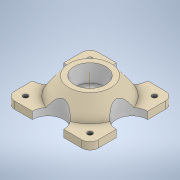
# Autodesk Inventor part: WindTurbine
Saved by Autodesk Inventor 2021 (Build 250183000, 183)
## iProperties
Created: 2022-01-11
Part Number: WindTurbine
Material: Generic
Document SubType Name: Modeling
Designer: stefi
Density: 1 g/cm^3
Appearance: Default
Author: stefi
Autodesk Inventor part; units mm, degrees
ref_plane "YZ Plane" through (0, 0, 0) normal (1, 0, 0) x (0, 1, 0)
ref_plane "XZ Plane" through (0, 0, 0) normal (0, 1, 0) x (-1, 0, 0)
ref_plane "XY Plane" through (0, 0, 0) normal (0, 0, 1) x (1, 0, 0)
sketch "Sketch1" plane through (0, 0, 0) normal (0, 1, 0) x (-1, 0, 0)
  line L0 (40.8, 50.8) -> (-40.8, 50.8)
  line L1 (-50.8, 40.8) -> (-50.8, -40.8)
  line L2 (-40.8, -50.8) -> (40.8, -50.8)
  line L3 (50.8, -40.8) -> (50.8, 40.8)
  line L4 (50.8, 50.8) -> (-50.8, -50.8) construction
  line L5 (-50.8, 50.8) -> (50.8, -50.8) construction
  arc A0 (50.8, 40.8) -> (40.8, 50.8) centre (40.8, 40.8) ccw
  arc A1 (-40.8, 50.8) -> (-50.8, 40.8) centre (-40.8, 40.8) ccw
  arc A2 (-50.8, -40.8) -> (-40.8, -50.8) centre (-40.8, -40.8) ccw
  arc A3 (40.8, -50.8) -> (50.8, -40.8) centre (40.8, -40.8) ccw
  point P0 (0, 0)
  dimension "d0" = 101.6
  dimension "d1" = 101.6
  dimension "d2" = 10
  constraints: 12 end point, 8 point on circle, 8 point on line, 8 tangent, 4 centre point, 3 equal radius, 2 midpoint, 2 parallel, 1 horizontal, 1 perpendicular
  measures "d0" distance of L5.end L4.end
  measures "d1" distance of L4.end L5.start
  measures "d2" radius of A0
extrude "Extrusion1" add sketch "Sketch1" along normal blind 8.8
sketch "Sketch2" plane through (0, 0, 0) normal (1, 0, 0) x (0, 1, 0)
  line L0 (8.8, 40.8) -> (8.8, -40.8) projected
  line L1 (8.8, 0) -> (30.3, 0)
  line L2 (30.3, 0) -> (30.3, -25.4)
  line L3 (30.3, -25.4) -> (8.8, -41.28)
  line L4 (8.8, 0) -> (8.8, -41.28)
  line L5 (-49.004, 0) -> (294.024, 0) projected
  point P0 (0, 0)
  dimension "d5" = 25.4
  dimension "d6" = 21.5
  dimension "d7" = 41.28
  constraints: 8 end point, 1 horizontal, 1 midpoint, 1 parallel, 1 perpendicular, 1 point on line
  measures "d5" distance of L1.end L2.end
  measures "d6" distance of L1.start L1.end
  measures "d7" distance of L3.end L1.start
revolve "Revolution1" add sketch "Sketch2" angle 360 about axis through (0, -10, 0) along (0, 1, 0)
sketch "Sketch3" plane through (0, 30.3, 0) normal (0, 1, 0) x (1, 0, 0)
  circle A0 centre (0, 0) radius 41.28 projected
  circle A1 centre (0, 0) radius 19.05
  line L0 (40.8, 50.8) -> (-40.8, 50.8) projected
  arc A2 (-19.05, 50.8) -> (19.05, 50.8) centre (0, 50.8) ccw
  line L1 (50.8, -40.8) -> (50.8, 40.8) projected
  arc A3 (50.8, 19.05) -> (50.8, -19.05) centre (50.8, 0) ccw
  line L2 (-40.8, -50.8) -> (40.8, -50.8) projected
  arc A4 (19.05, -50.8) -> (-19.05, -50.8) centre (0, -50.8) ccw
  line L3 (-50.8, 40.8) -> (-50.8, -40.8) projected
  arc A5 (-50.8, -19.05) -> (-50.8, 19.05) centre (-50.8, 0) ccw
  line L4 (-50.8, -19.05) -> (-50.8, 19.05)
  line L5 (-19.05, 50.8) -> (19.05, 50.8)
  line L6 (50.8, 19.05) -> (50.8, -19.05)
  line L7 (19.05, -50.8) -> (-19.05, -50.8)
  line L8 (-39.031, 39.031) -> (39.031, 39.031)
  line L9 (39.031, 39.031) -> (39.031, -39.031)
  line L10 (39.031, -39.031) -> (-39.031, -39.031)
  line L11 (-39.031, -39.031) -> (-39.031, 39.031)
  line L12 (-39.031, 39.031) -> (39.031, -39.031) construction
  line L13 (39.031, 39.031) -> (-39.031, -39.031) construction
  circle A6 centre (-39.031, 39.031) radius 3.0175
  circle A7 centre (39.031, 39.031) radius 3.0175
  circle A8 centre (39.031, -39.031) radius 3.0175
  circle A9 centre (-39.031, -39.031) radius 3.0175
  point P0 (50.8, 19.05)
  dimension "d9" = 38.1
  dimension "d10" = 78.062
  dimension "d11" = 78.062
  dimension "d12" = 6.035
  constraints: 20 end point, 9 centre point, 8 point on circle, 7 equal radius, 7 point on line, 6 midpoint, 5 coincident, 2 parallel, 1 horizontal, 1 perpendicular
  measures "d9" diameter of A5
  measures "d10" distance of L9.end L10.end
  measures "d11" distance of L8.end L9.end
  measures "d12" diameter of A6
extrude "Extrusion2" cut sketch "Sketch3" against normal through all contours A0 L9 | A0 L9 A3 L1 | L9 A0 A3 | A0 A3 L9 | L9 A3 A0 | A2 A0 L8 | A0 L8 A2 | A4 L10 A0 | A0 L10 A4 | L8 A0 | A0 L8 A2 L0 | A2 L8 A0 | L10 A4 L2 A0 | A0 L10 | A0 L10 A4 | A5 A0 L11 | A0 L11 A5 | A5 L11 A0 | L11 A0 | A0 L11 A5 L3 | A1
extrude "Extrusion3" cut sketch "Sketch3" against normal through all contours A7 L8 L9 | L9 L8 A7 | A8 L10 L9 | L9 L10 A8 | A6 L11 L8 | L8 L11 A6 | A9 L11 L10 | L10 L11 A9
sketch "Sketch4" plane through (0, 0, 0) normal (0, -1, 0) x (1, 0, 0)
  circle A0 centre (0, 0) radius 19.05
  dimension "d19" = 38.1
  constraints: 1 centre point, 1 coincident
  measures "d19" diameter of A0
extrude "Extrusion4" add sketch "Sketch4" against normal up to surface (8.8 mm away)
body "Solid1"
